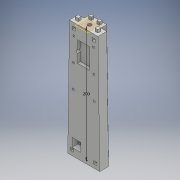
# Autodesk Inventor part: tb3_pt5
Saved by Autodesk Inventor 2017 (Build 210142000, 142)
## iProperties
Created: 2017-04-07
Part Number: tb3_pt5
Material: Generic
Document SubType Name: Modeling
Designer: PC
Density: 1 g/cm^3
Appearance: Default
Author: PC
Autodesk Inventor part; units mm, degrees
ref_plane "YZ Plane" through (0, 0, 0) normal (1, 0, 0) x (0, 1, 0)
ref_plane "XZ Plane" through (0, 0, 0) normal (0, 1, 0) x (-1, 0, 0)
ref_plane "XY Plane" through (0, 0, 0) normal (0, 0, 1) x (1, 0, 0)
sketch "Sketch1" plane through (0, 0, 0) normal (0, 0, 1) x (1, 0, 0)
  line L0 (27.5, -7.5) -> (-27.5, -7.5)
  line L1 (-27.5, -7.5) -> (-27.5, 7.5)
  line L2 (-27.5, 7.5) -> (27.5, 7.5)
  line L3 (27.5, 7.5) -> (27.5, -7.5)
  line L4 (27.5, -7.5) -> (-27.5, 7.5) construction
  line L5 (-27.5, -7.5) -> (27.5, 7.5) construction
  point P0 (0, 0)
  dimension "d0" = 55
  dimension "d1" = 15
  constraints: 12 end point, 2 midpoint, 2 parallel, 1 horizontal, 1 perpendicular
  measures "d0" distance of L1.end L2.end
  measures "d1" distance of L0.end L1.end
sketch "Sketch2" plane through (0, 0, 0) normal (0, 0, 1) x (1, 0, 0)
  line L0 (0, 0) -> (0, 12.5)
  line L1 (17.5, 17.5) -> (-17.5, 17.5)
  line L2 (-17.5, 17.5) -> (-17.5, 7.5)
  line L3 (-17.5, 7.5) -> (17.5, 7.5)
  line L4 (17.5, 7.5) -> (17.5, 17.5)
  line L5 (17.5, 17.5) -> (-17.5, 7.5) construction
  line L6 (-17.5, 17.5) -> (17.5, 7.5) construction
  dimension "d2" = 12.5
  dimension "d3" = 35
  dimension "d4" = 10
  constraints: 14 end point, 2 midpoint, 2 parallel, 1 horizontal, 1 perpendicular, 1 vertical
  measures "d2" distance of L0.start L0.end
  measures "d3" distance of L3.end L2.end
  measures "d4" distance of L2.end L1.end
sketch "Sketch3" plane through (0, 0, 0) normal (1, 0, 0) x (0, 1, 0)
  line L0 (0, 0) -> (0, 200)
  dimension "d5" = 200
  constraints: 2 end point, 1 vertical
  measures "d5" distance of L0.start L0.end
ref_plane "Work Plane1" through (0, 0, 200) normal (0, 0, 1) x (1, 0, 0)
sketch "Sketch4" plane through (0, 0, 200) normal (0, 0, 1) x (1, 0, 0)
  line L0 (24.5, -7.5) -> (-24.5, -7.5)
  line L1 (-24.5, -7.5) -> (-24.5, 7.5)
  line L2 (-24.5, 7.5) -> (24.5, 7.5)
  line L3 (24.5, 7.5) -> (24.5, -7.5)
  line L4 (24.5, -7.5) -> (-24.5, 7.5) construction
  line L5 (-24.5, -7.5) -> (24.5, 7.5) construction
  point P0 (0, 0)
  dimension "d6" = 49
  dimension "d7" = 15
  constraints: 12 end point, 2 midpoint, 2 parallel, 1 horizontal, 1 perpendicular
  measures "d6" distance of L1.end L2.end
  measures "d7" distance of L0.end L1.end
sketch "Sketch5" plane through (0, 0, 200) normal (0, 0, 1) x (1, 0, 0)
  line L0 (0, 0) -> (0, 12.5)
  line L1 (-14.5, 17.5) -> (14.5, 17.5)
  line L2 (14.5, 17.5) -> (14.5, 7.5)
  line L3 (14.5, 7.5) -> (-14.5, 7.5)
  line L4 (-14.5, 7.5) -> (-14.5, 17.5)
  line L5 (-14.5, 17.5) -> (14.5, 7.5) construction
  line L6 (14.5, 17.5) -> (-14.5, 7.5) construction
  dimension "d8" = 12.5
  dimension "d9" = 29
  dimension "d10" = 10
  constraints: 14 end point, 2 midpoint, 2 parallel, 1 horizontal, 1 perpendicular, 1 vertical
  measures "d8" distance of L0.start L0.end
  measures "d9" distance of L2.end L3.end
  measures "d10" distance of L1.end L2.end
loft "Loft1" add profiles "Sketch4", "Sketch1"
loft "Loft2" add profiles "Sketch5", "Sketch2"
sketch "Sketch9" plane through (27.5, -7.5, 0) normal (0, 0, -1) x (-1, 0, 0)
  line L0 (3, 0) -> (52, 0) projected
  line L1 (10, 15) -> (0, 15) projected
  line L2 (27.5, 0) -> (0, 0)
  line L3 (0, 0) -> (0, 15)
  line L4 (0, 15) -> (27.5, 15)
  line L5 (27.5, 15) -> (27.5, 0)
  line L6 (0, 15) -> (13.75, 15)
  line L7 (13.75, 15) -> (13.75, 0)
  line L8 (13.75, 0) -> (0, 0)
  line L9 (0, 0) -> (0, 15)
  line L10 (6.875, 0) -> (0, 0)
  line L11 (0, 0) -> (0, 15)
  line L12 (0, 15) -> (6.875, 15)
  line L13 (6.875, 15) -> (6.875, 0)
  line L14 (9.625, 4.75) -> (4.125, 4.75)
  line L15 (4.125, 4.75) -> (4.125, 10.25)
  line L16 (4.125, 10.25) -> (9.625, 10.25)
  line L17 (9.625, 10.25) -> (9.625, 4.75)
  line L18 (9.625, 4.75) -> (4.125, 10.25) construction
  line L19 (4.125, 4.75) -> (9.625, 10.25) construction
  point P0 (27.5, 7.5)
  point P1 (6.875, 7.5)
  dimension "d34" = 5.5
  dimension "d35" = 5.5
  constraints: 36 end point, 8 parallel, 6 midpoint, 4 horizontal, 4 perpendicular
  measures "d34" distance of L15.end L16.end
  measures "d35" distance of L14.end L15.end
sketch "Sketch10" plane through (27.5, -7.5, 0) normal (0, 0, -1) x (-1, 0, 0)
  line L0 (55, 0) -> (55, 15) projected
  line L1 (3, 0) -> (52, 0) projected
  line L2 (55, 15) -> (27.5, 15)
  line L3 (27.5, 15) -> (27.5, 0)
  line L4 (27.5, 0) -> (55, 0)
  line L5 (55, 0) -> (55, 15)
  line L6 (55, 15) -> (41.25, 15)
  line L7 (41.25, 15) -> (41.25, 0)
  line L8 (41.25, 0) -> (55, 0)
  line L9 (55, 0) -> (55, 15)
  line L10 (55, 15) -> (48.125, 15)
  line L11 (48.125, 15) -> (48.125, 0)
  line L12 (48.125, 0) -> (55, 0)
  line L13 (55, 0) -> (55, 15)
  line L14 (50.875, 4.75) -> (45.375, 4.75)
  line L15 (45.375, 4.75) -> (45.375, 10.25)
  line L16 (45.375, 10.25) -> (50.875, 10.25)
  line L17 (50.875, 10.25) -> (50.875, 4.75)
  line L18 (50.875, 4.75) -> (45.375, 10.25) construction
  line L19 (45.375, 4.75) -> (50.875, 10.25) construction
  point P0 (27.5, 7.5)
  point P1 (48.125, 7.5)
  dimension "d36" = 5.5
  dimension "d37" = 5.5
  constraints: 36 end point, 8 parallel, 6 midpoint, 4 horizontal, 4 perpendicular
  measures "d36" distance of L15.end L16.end
  measures "d37" distance of L14.end L15.end
sketch "Sketch13" plane through (-24.5, -7.5, 200) normal (0, 0, 1) x (1, 0, 0)
  line L0 (8.625, 5) -> (3.625, 10) construction
  line L1 (3.625, 5) -> (8.625, 10) construction
  line L2 (0, 0) -> (-3, 0) projected
  line L3 (0, 0) -> (5, 0)
  line L4 (5, 0) -> (5, 5)
  line L5 (5, 5) -> (0, 5)
  line L6 (0, 5) -> (0, 0)
  line L7 (5, 5) -> (10, 5)
  line L8 (10, 5) -> (10, 10)
  line L9 (10, 10) -> (5, 10)
  line L10 (5, 10) -> (5, 5)
  point P0 (24.5, 7.5)
  point P1 (0, 15)
  point P2 (6.125, 7.5)
  dimension "d296" = 5
  dimension "d297" = 5
  dimension "d298" = 5
  dimension "d299" = 5
  constraints: 20 end point, 4 parallel, 2 horizontal, 2 midpoint, 2 perpendicular
  measures "d296" distance of L5.end L4.end
  measures "d297" distance of L4.end L3.end
  measures "d298" distance of L9.end L8.end
  measures "d299" distance of L8.end L7.end
sketch "Sketch14" plane through (-24.5, -7.5, 200) normal (0, 0, 1) x (1, 0, 0)
  line L0 (45.375, 5) -> (40.375, 10) construction
  line L1 (40.375, 5) -> (45.375, 10) construction
  line L2 (49, 0) -> (52, 0) projected
  line L3 (49, 0) -> (44, 0)
  line L4 (44, 0) -> (44, 5)
  line L5 (44, 5) -> (49, 5)
  line L6 (49, 5) -> (49, 0)
  line L7 (44, 5) -> (39, 5)
  line L8 (39, 5) -> (39, 10)
  line L9 (39, 10) -> (44, 10)
  line L10 (44, 10) -> (44, 5)
  point P0 (24.5, 7.5)
  point P1 (49, 15)
  point P2 (42.875, 7.5)
  dimension "d302" = 5
  dimension "d303" = 5
  dimension "d304" = 5
  dimension "d305" = 5
  constraints: 20 end point, 4 parallel, 2 horizontal, 2 midpoint, 2 perpendicular
  measures "d302" distance of L4.end L5.end
  measures "d303" distance of L3.end L4.end
  measures "d304" distance of L8.end L9.end
  measures "d305" distance of L7.end L8.end
extrude "Extrusion9" cut sketch "Sketch9" against normal blind 6 contours L14 L15 L16 L13 | L13 L16 L17 L14
extrude "Extrusion12" cut sketch "Sketch10" against normal blind 6 contours L16 L17 L14 L11 | L11 L14 L15 L16
sketch "Sketch18" plane through (14.5, 7.5, 200) normal (0, 1, 0) x (1, 0, 0)
  line L0 (3, 200) -> (0, 0) projected
  line L1 (1.5, 100) -> (3.5, 100)
  line L2 (2.9, 100.6) -> (4.1, 100.6)
  line L3 (4.1, 100.6) -> (4.1, 99.4)
  line L4 (4.1, 99.4) -> (2.9, 99.4)
  line L5 (2.9, 99.4) -> (2.9, 100.6)
  line L6 (2.9, 100.6) -> (4.1, 99.4) construction
  line L7 (4.1, 100.6) -> (2.9, 99.4) construction
  point P0 (-14.5, 200)
  dimension "d90" = 2
  dimension "d103" = 1.2
  dimension "d104" = 1.2
  constraints: 14 end point, 3 midpoint, 2 horizontal, 2 parallel, 1 perpendicular
  measures "d90" distance of L1.start L1.end
  measures "d103" distance of L3.end L4.end
  measures "d104" distance of L2.end L3.end
sketch "Sketch19" plane through (14.5, 7.5, 200) normal (0, 1, 0) x (1, 0, 0)
  line L0 (3, 200) -> (0, 0) projected
  line L1 (0.9, 60) -> (2.9, 60)
  line L2 (0.9, 60) -> (2.9, 60) construction
  line L3 (2.3, 60.6) -> (3.5, 60.6)
  line L4 (3.5, 60.6) -> (3.5, 59.4)
  line L5 (3.5, 59.4) -> (2.3, 59.4)
  line L6 (2.3, 59.4) -> (2.3, 60.6)
  line L7 (2.3, 60.6) -> (3.5, 59.4) construction
  line L8 (3.5, 60.6) -> (2.3, 59.4) construction
  point P0 (-14.5, 200)
  dimension "d91" = 2
  dimension "d92" = 0
  dimension "d111" = 1.2
  dimension "d112" = 1.2
  constraints: 16 end point, 3 horizontal, 2 midpoint, 2 parallel, 1 collinear, 1 perpendicular, 1 point on line
  measures "d91" distance of L1.start L1.end
  measures "d92" distance between parallel lines of L1 L2
  measures "d111" distance of L4.end L5.end
  measures "d112" distance of L3.end L4.end
sketch "Sketch20" plane through (14.5, 7.5, 200) normal (0, 1, 0) x (1, 0, 0)
  line L0 (3, 200) -> (0, 0) projected
  line L1 (0.3, 20) -> (2.3, 20)
  line L2 (0.3, 20) -> (2.3, 20) construction
  line L3 (1.7, 20.6) -> (2.9, 20.6)
  line L4 (2.9, 20.6) -> (2.9, 19.4)
  line L5 (2.9, 19.4) -> (1.7, 19.4)
  line L6 (1.7, 19.4) -> (1.7, 20.6)
  line L7 (1.7, 20.6) -> (2.9, 19.4) construction
  line L8 (2.9, 20.6) -> (1.7, 19.4) construction
  point P0 (-14.5, 200)
  dimension "d93" = 2
  dimension "d94" = 0
  dimension "d119" = 1.2
  dimension "d120" = 1.2
  constraints: 16 end point, 3 horizontal, 2 midpoint, 2 parallel, 1 collinear, 1 perpendicular, 1 point on line
  measures "d93" distance of L1.start L1.end
  measures "d94" distance between parallel lines of L1 L2
  measures "d119" distance of L4.end L5.end
  measures "d120" distance of L3.end L4.end
extrude "Extrusion21" cut sketch "Sketch18" against normal blind 6.6
sketch "Sketch22" plane through (14.5, 0.9, 200) normal (0, 1, 0) x (1, 0, 0)
  line L0 (2.1, 101.4) -> (4.9, 101.4)
  line L1 (4.9, 101.4) -> (4.9, 98.6)
  line L2 (4.9, 98.6) -> (2.1, 98.6)
  line L3 (2.1, 98.6) -> (2.1, 101.4)
  line L4 (2.1, 101.4) -> (4.9, 98.6) construction
  line L5 (4.9, 101.4) -> (2.1, 98.6) construction
  point P0 (-14.5, 200)
  point P1 (3.5, 100)
  dimension "d107" = 2.8
  dimension "d108" = 2.8
  constraints: 12 end point, 2 midpoint, 2 parallel, 1 horizontal, 1 perpendicular
  measures "d107" distance of L1.end L2.end
  measures "d108" distance of L0.end L1.end
extrude "Extrusion22" cut sketch "Sketch22" against normal through all
extrude "Extrusion23" cut sketch "Sketch19" against normal blind 6.6
sketch "Sketch23" plane through (14.5, 0.9, 200) normal (0, 1, 0) x (1, 0, 0)
  line L0 (1.5, 61.4) -> (4.3, 61.4)
  line L1 (4.3, 61.4) -> (4.3, 58.6)
  line L2 (4.3, 58.6) -> (1.5, 58.6)
  line L3 (1.5, 58.6) -> (1.5, 61.4)
  line L4 (1.5, 61.4) -> (4.3, 58.6) construction
  line L5 (4.3, 61.4) -> (1.5, 58.6) construction
  point P0 (-14.5, 200)
  point P1 (2.9, 60)
  dimension "d115" = 2.8
  dimension "d116" = 2.8
  constraints: 12 end point, 2 midpoint, 2 parallel, 1 horizontal, 1 perpendicular
  measures "d115" distance of L1.end L2.end
  measures "d116" distance of L0.end L1.end
extrude "Extrusion24" cut sketch "Sketch23" against normal through all
extrude "Extrusion25" cut sketch "Sketch20" against normal blind 6.6
sketch "Sketch24" plane through (14.5, 0.9, 200) normal (0, 1, 0) x (1, 0, 0)
  line L0 (0.9, 21.4) -> (3.7, 21.4)
  line L1 (3.7, 21.4) -> (3.7, 18.6)
  line L2 (3.7, 18.6) -> (0.9, 18.6)
  line L3 (0.9, 18.6) -> (0.9, 21.4)
  line L4 (0.9, 21.4) -> (3.7, 18.6) construction
  line L5 (3.7, 21.4) -> (0.9, 18.6) construction
  point P0 (-14.5, 200)
  point P1 (2.3, 20)
  dimension "d123" = 2.8
  dimension "d124" = 2.8
  constraints: 12 end point, 2 midpoint, 2 parallel, 1 horizontal, 1 perpendicular
  measures "d123" distance of L1.end L2.end
  measures "d124" distance of L0.end L1.end
extrude "Extrusion26" cut sketch "Sketch24" against normal through all
sketch "Sketch30" plane through (-27.5, 7.5, 0) normal (0, 1, 0) x (1, 0, 0)
  line L0 (13, -200) -> (10, 0) projected
  line L1 (11.5, -100) -> (9.5, -100)
  line L2 (10.1, -99.4) -> (8.9, -99.4)
  line L3 (8.9, -99.4) -> (8.9, -100.6)
  line L4 (8.9, -100.6) -> (10.1, -100.6)
  line L5 (10.1, -100.6) -> (10.1, -99.4)
  line L6 (10.1, -99.4) -> (8.9, -100.6) construction
  line L7 (8.9, -99.4) -> (10.1, -100.6) construction
  point P0 (27.5, 0)
  dimension "d147" = 2
  dimension "d148" = 1.2
  dimension "d149" = 1.2
  constraints: 14 end point, 3 midpoint, 2 horizontal, 2 parallel, 1 perpendicular
  measures "d147" distance of L1.start L1.end
  measures "d148" distance of L4.end L3.end
  measures "d149" distance of L3.end L2.end
extrude "Extrusion31" cut sketch "Sketch30" against normal blind 6.6
sketch "Sketch31" plane through (-27.5, 0.9, 0) normal (0, 1, 0) x (1, 0, 0)
  line L0 (8.1, -98.6) -> (10.9, -98.6)
  line L1 (10.9, -98.6) -> (10.9, -101.4)
  line L2 (10.9, -101.4) -> (8.1, -101.4)
  line L3 (8.1, -101.4) -> (8.1, -98.6)
  line L4 (8.1, -98.6) -> (10.9, -101.4) construction
  line L5 (10.9, -98.6) -> (8.1, -101.4) construction
  point P0 (27.5, 0)
  point P1 (9.5, -100)
  dimension "d152" = 2.8
  dimension "d153" = 2.8
  constraints: 12 end point, 2 midpoint, 2 parallel, 1 horizontal, 1 perpendicular
  measures "d152" distance of L1.end L2.end
  measures "d153" distance of L0.end L1.end
extrude "Extrusion32" cut sketch "Sketch31" against normal through all
sketch "Sketch32" plane through (-27.5, 7.5, 0) normal (0, 1, 0) x (1, 0, 0)
  line L0 (13, -200) -> (10, 0) projected
  line L1 (12.1, -140) -> (10.1, -140)
  line L2 (12.1, -140) -> (14.1, -140) construction
  line L3 (10.7, -139.4) -> (9.5, -139.4)
  line L4 (9.5, -139.4) -> (9.5, -140.6)
  line L5 (9.5, -140.6) -> (10.7, -140.6)
  line L6 (10.7, -140.6) -> (10.7, -139.4)
  line L7 (10.7, -139.4) -> (9.5, -140.6) construction
  line L8 (9.5, -139.4) -> (10.7, -140.6) construction
  point P0 (27.5, 0)
  dimension "d156" = 2
  dimension "d157" = 180
  dimension "d158" = 1.2
  dimension "d159" = 1.2
  constraints: 16 end point, 3 horizontal, 2 midpoint, 2 parallel, 1 collinear, 1 perpendicular, 1 point on line
  measures "d156" distance of L1.start L1.end
  measures "d157" angle of L1 L2
  measures "d158" distance of L5.end L4.end
  measures "d159" distance of L4.end L3.end
extrude "Extrusion33" cut sketch "Sketch32" against normal blind 6.6
sketch "Sketch33" plane through (-27.5, 0.9, 0) normal (0, 1, 0) x (1, 0, 0)
  line L0 (8.7, -138.6) -> (11.5, -138.6)
  line L1 (11.5, -138.6) -> (11.5, -141.4)
  line L2 (11.5, -141.4) -> (8.7, -141.4)
  line L3 (8.7, -141.4) -> (8.7, -138.6)
  line L4 (8.7, -138.6) -> (11.5, -141.4) construction
  line L5 (11.5, -138.6) -> (8.7, -141.4) construction
  point P0 (27.5, 0)
  point P1 (10.1, -140)
  dimension "d162" = 2.8
  dimension "d163" = 2.8
  constraints: 12 end point, 2 midpoint, 2 parallel, 1 horizontal, 1 perpendicular
  measures "d162" distance of L1.end L2.end
  measures "d163" distance of L0.end L1.end
extrude "Extrusion34" cut sketch "Sketch33" against normal through all
sketch "Sketch34" plane through (-27.5, 7.5, 0) normal (0, 1, 0) x (1, 0, 0)
  line L0 (13, -200) -> (10, 0) projected
  line L1 (12.7, -180) -> (10.7, -180)
  line L2 (12.7, -180) -> (14.7, -180) construction
  line L3 (10.1, -179.4) -> (11.3, -179.4)
  line L4 (11.3, -179.4) -> (11.3, -180.6)
  line L5 (11.3, -180.6) -> (10.1, -180.6)
  line L6 (10.1, -180.6) -> (10.1, -179.4)
  line L7 (10.1, -179.4) -> (11.3, -180.6) construction
  line L8 (11.3, -179.4) -> (10.1, -180.6) construction
  point P0 (27.5, 0)
  dimension "d166" = 2
  dimension "d167" = 180
  dimension "d168" = 1.2
  dimension "d169" = 1.2
  constraints: 16 end point, 3 horizontal, 2 midpoint, 2 parallel, 1 collinear, 1 perpendicular, 1 point on line
  measures "d166" distance of L1.start L1.end
  measures "d167" angle of L1 L2
  measures "d168" distance of L4.end L5.end
  measures "d169" distance of L3.end L4.end
extrude "Extrusion35" cut sketch "Sketch34" against normal blind 6.6
sketch "Sketch35" plane through (-27.5, 0.9, 0) normal (0, 1, 0) x (1, 0, 0)
  line L0 (9.3, -178.6) -> (12.1, -178.6)
  line L1 (12.1, -178.6) -> (12.1, -181.4)
  line L2 (12.1, -181.4) -> (9.3, -181.4)
  line L3 (9.3, -181.4) -> (9.3, -178.6)
  line L4 (9.3, -178.6) -> (12.1, -181.4) construction
  line L5 (12.1, -178.6) -> (9.3, -181.4) construction
  point P0 (27.5, 0)
  point P1 (10.7, -180)
  dimension "d172" = 2.8
  dimension "d173" = 2.8
  constraints: 12 end point, 2 midpoint, 2 parallel, 1 horizontal, 1 perpendicular
  measures "d172" distance of L1.end L2.end
  measures "d173" distance of L0.end L1.end
extrude "Extrusion36" cut sketch "Sketch35" against normal through all
chamfer "Chamfer3" distance 0.8 angle 45 4 edges at (-18, 0.9, 100.6) (-18.6, 0.9, 100) (-18, 0.9, 99.4) (-17.4, 0.9, 100)
chamfer "Chamfer4" distance 0.8 angle 45 4 edges at (-18, 0.9, 140) (-17.4, 0.9, 140.6) (-16.8, 0.9, 140) (-17.4, 0.9, 139.4)
chamfer "Chamfer5" distance 0.8 angle 45 4 edges at (-16.8, 0.9, 180.6) (-17.4, 0.9, 180) (-16.8, 0.9, 179.4) (-16.2, 0.9, 180)
chamfer "Chamfer8" distance 0.8 angle 45 4 edges at (17.4, 0.9, 100) (18, 0.9, 100.6) (18.6, 0.9, 100) (18, 0.9, 99.4)
chamfer "Chamfer9" distance 0.8 angle 45 4 edges at (16.8, 0.9, 140) (17.4, 0.9, 140.6) (18, 0.9, 140) (17.4, 0.9, 139.4)
chamfer "Chamfer10" distance 0.8 angle 45 4 edges at (16.2, 0.9, 180) (16.8, 0.9, 180.6) (17.4, 0.9, 180) (16.8, 0.9, 179.4)
sketch "Sketch38" plane through (-27.5, -7.5, 0) normal (0, -1, 0) x (1, 0, 0)
  line L0 (12.5, 22.5) -> (17.5, 22.5)
  line L1 (17.5, 22.5) -> (17.5, 17.5)
  line L2 (17.5, 17.5) -> (12.5, 17.5)
  line L3 (12.5, 17.5) -> (12.5, 22.5)
  line L4 (12.5, 22.5) -> (17.5, 17.5) construction
  line L5 (17.5, 22.5) -> (12.5, 17.5) construction
  point P0 (27.5, 0)
  point P1 (15, 20)
  dimension "d210" = 5
  dimension "d211" = 5
  constraints: 12 end point, 2 midpoint, 2 parallel, 1 horizontal, 1 perpendicular
  measures "d210" distance of L1.end L2.end
  measures "d211" distance of L0.end L1.end
extrude "Extrusion37" cut sketch "Sketch38" against normal blind 5
chamfer "Chamfer11" distance 5 angle 45 4 edges at (-12.5, -7.5, 17.5) (-15, -7.5, 20) (-10, -7.5, 20) (-12.5, -7.5, 22.5)
sketch "Sketch40" plane through (-17.5, 17.5, 0) normal (0, 1, 0) x (1, 0, 0)
  line L0 (17.5, 0) -> (17.5, -20)
  line L1 (17.5, -20) -> (5, -20)
  line L2 (4.4, -20.6) -> (5.6, -20.6)
  line L3 (5.6, -20.6) -> (5.6, -19.4)
  line L4 (5.6, -19.4) -> (4.4, -19.4)
  line L5 (4.4, -19.4) -> (4.4, -20.6)
  line L6 (4.4, -20.6) -> (5.6, -19.4) construction
  line L7 (5.6, -20.6) -> (4.4, -19.4) construction
  dimension "d217" = 12.5
  dimension "d218" = 1.2
  dimension "d219" = 1.2
  constraints: 16 end point, 2 midpoint, 2 parallel, 2 perpendicular, 1 horizontal, 1 vertical
  measures "d217" distance of L0.end L1.end
  measures "d218" distance of L4.end L3.end
  measures "d219" distance of L3.end L2.end
extrude "Extrusion38" cut sketch "Sketch40" against normal blind 7.8
sketch "Sketch41" plane through (-17.5, 9.7, 0) normal (0, 1, 0) x (1, 0, 0)
  line L0 (6.4, -21.4) -> (3.6, -21.4)
  line L1 (3.6, -21.4) -> (3.6, -18.6)
  line L2 (3.6, -18.6) -> (6.4, -18.6)
  line L3 (6.4, -18.6) -> (6.4, -21.4)
  line L4 (6.4, -21.4) -> (3.6, -18.6) construction
  line L5 (3.6, -21.4) -> (6.4, -18.6) construction
  point P0 (17.5, 0)
  point P1 (5, -20)
  dimension "d222" = 2.8
  dimension "d223" = 2.8
  constraints: 12 end point, 2 midpoint, 2 parallel, 1 horizontal, 1 perpendicular
  measures "d222" distance of L1.end L2.end
  measures "d223" distance of L0.end L1.end
extrude "Extrusion39" cut sketch "Sketch41" against normal through all
chamfer "Chamfer12" distance 0.8 angle 45 4 edges at (-12.5, 9.7, 19.4) (-11.9, 9.7, 20) (-12.5, 9.7, 20.6) (-13.1, 9.7, 20)
sketch "Sketch42" plane through (27.5, -7.5, 0) normal (0, 0, -1) x (-1, 0, 0)
  line L0 (27.5, 25) -> (27.5, 10)
  point P0 (27.5, 7.5)
  dimension "d229" = 15
  constraints: 2 end point, 1 vertical
  measures "d229" distance of L0.start L0.end
hole "Hole2" at (0, 2.5, 0) direction (0, 0, 1) diameter 6.4 end through all
sketch "Sketch44" plane through (-27.5, -7.5, 0) normal (0, -1, 0) x (1, 0, 0)
  line L0 (38, 142.5) -> (17, 142.5)
  line L1 (17, 142.5) -> (17, 177.5)
  line L2 (17, 177.5) -> (38, 177.5)
  line L3 (38, 177.5) -> (38, 142.5)
  line L4 (38, 142.5) -> (17, 177.5) construction
  line L5 (17, 142.5) -> (38, 177.5) construction
  point P0 (27.5, 0)
  point P1 (27.5, 160)
  dimension "d237" = 21
  dimension "d238" = 35
  constraints: 12 end point, 2 midpoint, 2 parallel, 1 horizontal, 1 perpendicular
  measures "d237" distance of L1.end L2.end
  measures "d238" distance of L0.end L1.end
extrude "Extrusion40" cut sketch "Sketch44" against normal blind 5
sketch "Sketch46" plane through (-27.5, -7.5, 0) normal (0, -1, 0) x (1, 0, 0)
  line L0 (55, 0) -> (47.5, 0)
  line L1 (47.5, 0) -> (47.5, 9)
  line L2 (47.5, 9) -> (55, 9)
  line L3 (55, 9) -> (55, 0)
  line L4 (45, 11.5) -> (50, 11.5)
  line L5 (50, 11.5) -> (50, 6.5)
  line L6 (50, 6.5) -> (45, 6.5)
  line L7 (45, 6.5) -> (45, 11.5)
  line L8 (45, 11.5) -> (50, 6.5) construction
  line L9 (50, 11.5) -> (45, 6.5) construction
  point P0 (27.5, 0)
  dimension "d241" = 7.5
  dimension "d242" = 9
  dimension "d243" = 5
  dimension "d244" = 5
  constraints: 20 end point, 4 parallel, 2 horizontal, 2 midpoint, 2 perpendicular
  measures "d241" distance of L1.end L2.end
  measures "d242" distance of L0.end L1.end
  measures "d243" distance of L5.end L6.end
  measures "d244" distance of L4.end L5.end
sketch "Sketch47" plane through (-27.5, -7.5, 0) normal (0, -1, 0) x (1, 0, 0)
  line L0 (0, 0) -> (7.5, 0)
  line L1 (7.5, 0) -> (7.5, 9)
  line L2 (7.5, 9) -> (0, 9)
  line L3 (0, 9) -> (0, 0)
  line L4 (10, 11.5) -> (5, 11.5)
  line L5 (5, 11.5) -> (5, 6.5)
  line L6 (5, 6.5) -> (10, 6.5)
  line L7 (10, 6.5) -> (10, 11.5)
  line L8 (10, 11.5) -> (5, 6.5) construction
  line L9 (5, 11.5) -> (10, 6.5) construction
  point P0 (27.5, 0)
  dimension "d245" = 7.5
  dimension "d246" = 9
  dimension "d247" = 5
  dimension "d248" = 5
  constraints: 20 end point, 4 parallel, 2 horizontal, 2 midpoint, 2 perpendicular
  measures "d245" distance of L2.end L1.end
  measures "d246" distance of L1.end L0.end
  measures "d247" distance of L6.end L5.end
  measures "d248" distance of L5.end L4.end
sketch "Sketch48" plane through (-27.5, -7.5, 0) normal (0, -1, 0) x (1, 0, 0)
  line L0 (52, 200) -> (3, 200) projected
  line L1 (52, 200) -> (44.5, 200)
  line L2 (44.5, 200) -> (44.5, 191)
  line L3 (44.5, 191) -> (52, 191)
  line L4 (52, 191) -> (52, 200)
  line L5 (42, 193.5) -> (47, 193.5)
  line L6 (47, 193.5) -> (47, 188.5)
  line L7 (47, 188.5) -> (42, 188.5)
  line L8 (42, 188.5) -> (42, 193.5)
  line L9 (42, 193.5) -> (47, 188.5) construction
  line L10 (47, 193.5) -> (42, 188.5) construction
  line L11 (3, 200) -> (10.5, 200)
  line L12 (10.5, 200) -> (10.5, 191)
  line L13 (10.5, 191) -> (3, 191)
  line L14 (3, 191) -> (3, 200)
  line L15 (8, 193.5) -> (13, 193.5)
  line L16 (13, 193.5) -> (13, 188.5)
  line L17 (13, 188.5) -> (8, 188.5)
  line L18 (8, 188.5) -> (8, 193.5)
  line L19 (8, 193.5) -> (13, 188.5) construction
  line L20 (13, 193.5) -> (8, 188.5) construction
  point P0 (27.5, 0)
  dimension "d249" = 7.5
  dimension "d250" = 9
  dimension "d251" = 5
  dimension "d252" = 5
  dimension "d253" = 7.5
  dimension "d254" = 9
  dimension "d255" = 5
  dimension "d256" = 5
  constraints: 40 end point, 8 parallel, 4 horizontal, 4 midpoint, 4 perpendicular
  measures "d249" distance of L3.end L2.end
  measures "d250" distance of L2.end L1.end
  measures "d251" distance of L6.end L7.end
  measures "d252" distance of L5.end L6.end
  measures "d253" distance of L12.end L13.end
  measures "d254" distance of L11.end L12.end
  measures "d255" distance of L16.end L17.end
  measures "d256" distance of L15.end L16.end
extrude "Extrusion41" cut sketch "Sketch48" against normal blind 6 contours L5 L6 L3 L2 | L2 L3 L6 L7 L8 L5
extrude "Extrusion42" cut sketch "Sketch46" against normal blind 6 contours L6 L7 L4 L5 L2 L1 | L1 L2 L5 L6
extrude "Extrusion43" cut sketch "Sketch47" against normal blind 6 contours L6 L5 L2 L1 | L1 L2 L5 L4 L7 L6
sketch "Sketch49" plane through (-27.5, -7.5, 0) normal (0, -1, 0) x (1, 0, 0)
  line L0 (52, 200) -> (3, 200) projected
  line L1 (3, 200) -> (10.5, 200)
  line L2 (10.5, 200) -> (10.5, 191)
  line L3 (10.5, 191) -> (3, 191)
  line L4 (3, 191) -> (3, 200)
  line L5 (13, 188.5) -> (8, 188.5)
  line L6 (8, 188.5) -> (8, 193.5)
  line L7 (8, 193.5) -> (13, 193.5)
  line L8 (13, 193.5) -> (13, 188.5)
  line L9 (13, 188.5) -> (8, 193.5) construction
  line L10 (8, 188.5) -> (13, 193.5) construction
  point P0 (27.5, 0)
  dimension "d263" = 7.5
  dimension "d264" = 9
  dimension "d265" = 5
  dimension "d266" = 5
  constraints: 20 end point, 4 parallel, 2 horizontal, 2 midpoint, 2 perpendicular
  measures "d263" distance of L2.end L3.end
  measures "d264" distance of L1.end L2.end
  measures "d265" distance of L6.end L7.end
  measures "d266" distance of L5.end L6.end
extrude "Extrusion44" cut sketch "Sketch49" against normal blind 6 contours L7 L8 L5 L6 L3 L2 | L2 L3 L6 L7
sketch "Sketch51" plane through (-27.5, -7.5, 0) normal (0, -1, 0) x (1, 0, 0)
  line L0 (17, 142.5) -> (17, 177.5) projected
  circle A0 centre (17, 160) radius 2.5
  point P0 (27.5, 0)
  dimension "d269" = 5
  constraints: 1 centre point, 1 midpoint
  measures "d269" diameter of A0
extrude "Extrusion45" cut sketch "Sketch51" against normal blind 5
sketch "Sketch52" plane through (-24.5, -7.5, 200) normal (0, 0, 1) x (1, 0, 0)
  line L0 (39, 25) -> (42, 25) projected
  line L1 (39, 25) -> (24.5, 25)
  line L2 (24.5, 25) -> (24.5, 15)
  line L3 (24.5, 15) -> (39, 15)
  line L4 (39, 15) -> (39, 25)
  line L5 (39, 25) -> (31.75, 25)
  line L6 (31.75, 25) -> (31.75, 15)
  line L7 (31.75, 15) -> (39, 15)
  line L8 (39, 15) -> (39, 25)
  line L9 (29.5, 22.25) -> (34, 22.25)
  line L10 (34, 22.25) -> (34, 17.75)
  line L11 (34, 17.75) -> (29.5, 17.75)
  line L12 (29.5, 17.75) -> (29.5, 22.25)
  line L13 (29.5, 22.25) -> (34, 17.75) construction
  line L14 (34, 22.25) -> (29.5, 17.75) construction
  point P0 (24.5, 7.5)
  point P1 (31.75, 20)
  dimension "d312" = 4.5
  dimension "d313" = 4.5
  constraints: 28 end point, 6 parallel, 4 midpoint, 3 horizontal, 3 perpendicular
  measures "d312" distance of L10.end L11.end
  measures "d313" distance of L9.end L10.end
sketch "Sketch53" plane through (-24.5, -7.5, 200) normal (0, 0, 1) x (1, 0, 0)
  line L0 (10, 25) -> (15, 25)
  line L1 (10, 25) -> (24.5, 25)
  line L2 (24.5, 25) -> (24.5, 15)
  line L3 (24.5, 15) -> (10, 15)
  line L4 (10, 15) -> (10, 25)
  line L5 (10, 25) -> (17.25, 25)
  line L6 (17.25, 25) -> (17.25, 15)
  line L7 (17.25, 15) -> (10, 15)
  line L8 (10, 15) -> (10, 25)
  line L9 (19.5, 17.75) -> (15, 17.75)
  line L10 (15, 17.75) -> (15, 22.25)
  line L11 (15, 22.25) -> (19.5, 22.25)
  line L12 (19.5, 22.25) -> (19.5, 17.75)
  line L13 (19.5, 17.75) -> (15, 22.25) construction
  line L14 (15, 17.75) -> (19.5, 22.25) construction
  point P0 (24.5, 7.5)
  point P1 (17.25, 20)
  dimension "d308" = 4.5
  dimension "d309" = 4.5
  constraints: 30 end point, 6 parallel, 4 horizontal, 4 midpoint, 3 perpendicular
  measures "d308" distance of L10.end L11.end
  measures "d309" distance of L9.end L10.end
sketch "Sketch54" plane through (27.5, -7.5, 0) normal (0, 0, -1) x (-1, 0, 0)
  line L0 (45, 25) -> (10, 25) projected
  line L1 (45, 25) -> (40.25, 25)
  line L2 (40.25, 25) -> (40.25, 20.25)
  line L3 (40.25, 20.25) -> (45, 20.25)
  line L4 (45, 20.25) -> (45, 25)
  line L5 (40.25, 20.25) -> (34.75, 20.25)
  line L6 (34.75, 20.25) -> (34.75, 14.75)
  line L7 (34.75, 14.75) -> (40.25, 14.75)
  line L8 (40.25, 14.75) -> (40.25, 20.25)
  point P0 (27.5, 7.5)
  dimension "d284" = 4.75
  dimension "d285" = 4.75
  dimension "d286" = 5.5
  dimension "d287" = 5.5
  constraints: 16 end point, 4 parallel, 2 horizontal, 2 perpendicular
  measures "d284" distance of L3.end L2.end
  measures "d285" distance of L2.end L1.end
  measures "d286" distance of L7.end L6.end
  measures "d287" distance of L6.end L5.end
extrude "Extrusion48" cut sketch "Sketch54" against normal blind 6 contours L8 L7 L6 L5
sketch "Sketch55" plane through (27.5, -7.5, 0) normal (0, 0, -1) x (-1, 0, 0)
  line L0 (10, 25) -> (10, 15) projected
  line L1 (10, 25) -> (14.75, 25)
  line L2 (14.75, 25) -> (14.75, 20.25)
  line L3 (14.75, 20.25) -> (10, 20.25)
  line L4 (10, 20.25) -> (10, 25)
  line L5 (14.75, 20.25) -> (20.25, 20.25)
  line L6 (20.25, 20.25) -> (20.25, 14.75)
  line L7 (20.25, 14.75) -> (14.75, 14.75)
  line L8 (14.75, 14.75) -> (14.75, 20.25)
  point P0 (27.5, 7.5)
  dimension "d290" = 4.75
  dimension "d291" = 4.75
  dimension "d292" = 5.5
  dimension "d293" = 5.5
  constraints: 16 end point, 4 parallel, 2 horizontal, 2 perpendicular
  measures "d290" distance of L2.end L3.end
  measures "d291" distance of L1.end L2.end
  measures "d292" distance of L6.end L7.end
  measures "d293" distance of L5.end L6.end
extrude "Extrusion49" cut sketch "Sketch55" against normal blind 6 contours L5 L6 L7 L8
extrude "Extrusion50" add sketch "Sketch13" along normal blind 5 contours L10 L9 L8 L7
extrude "Extrusion51" add sketch "Sketch14" along normal blind 5 contours L7 L8 L9 L10
extrude "Extrusion52" add sketch "Sketch53" along normal blind 5 contours L11 L12 L9 L6 | L6 L9 L10 L11
extrude "Extrusion53" add sketch "Sketch52" along normal blind 5 contours L9 L10 L11 L6 | L6 L11 L12 L9
body "Solid1"
